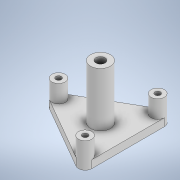
# Autodesk Inventor part: wheel_block
Saved by Autodesk Inventor 2021.3 (Build 253353010, 353A)
## iProperties
Created: 2021-11-06
Part Number: wheel_block
Material: Generic
Document SubType Name: Modeling
Designer: jesse
Density: 1 g/cm^3
Appearance: Default
Author: jesse
Autodesk Inventor part; units mm, degrees
ref_plane "YZ Plane" through (0, 0, 0) normal (1, 0, 0) x (0, 1, 0)
ref_plane "XZ Plane" through (0, 0, 0) normal (0, 1, 0) x (-1, 0, 0)
ref_plane "XY Plane" through (0, 0, 0) normal (0, 0, 1) x (1, 0, 0)
sketch "Sketch1" plane through (0, 0, 0) normal (0, 1, 0) x (-1, 0, 0)
  line L0 (27.1355, 0) -> (-13.5677, -23.5)
  line L1 (-13.5677, -23.5) -> (-13.5677, 23.5)
  line L2 (-13.5677, 23.5) -> (27.1355, 0)
  circle A0 centre (27.1355, 0) radius 1.8
  circle A1 centre (-13.5677, -23.5) radius 1.8
  circle A2 centre (-13.5677, 23.5) radius 1.8
  circle A3 centre (-13.5677, 23.5) radius 4.3
  circle A4 centre (-13.5677, -23.5) radius 4.3
  circle A5 centre (27.1355, 0) radius 4.3
  line L3 (37.2914, 0.8983) -> (-23.0689, -33.9507)
  line L4 (-17.8677, 35.8999) -> (-17.8677, -40.3839)
  line L5 (38.4842, -1.587) -> (-21.5839, 33.0933)
  point P0 (0, 0)
  point P1 (0, 0)
  point P2 (-11.4177, -27.2239)
  point P3 (29.2855, -3.7239)
  point P4 (29.2855, 3.7239)
  point P5 (-11.4177, 27.2239)
  point P6 (-17.8677, 23.5)
  point P7 (-17.8677, -23.5)
  dimension "d0" = 47
  dimension "d1" = 3.6
  dimension "d2" = 3.6
  dimension "d3" = 3.6
  dimension "d4" = 8.6
  dimension "d5" = 8.6
  dimension "d6" = 8.6
  constraints: 12 end point, 7 coincident, 6 centre point, 6 tangent, 7 other
  measures "d0" distance of L0.end L1.end
  measures "d1" diameter of A0
  measures "d2" diameter of A1
  measures "d3" diameter of A2
  measures "d4" diameter of A3
  measures "d5" diameter of A4
  measures "d6" diameter of A5
extrude "Extrusion1" add sketch "Sketch1" along normal blind 5 contours A0 L2 A5 L0 | L0 A5 L2 A0 | A5 L3 A4 L0 | L0 A4 L1 A3 L2 A5 | L2 A3 L5 A5 | A4 L1 A1 L0 | L0 A1 L1 A4 | A3 L1 A2 L2 | L2 A2 L1 A3 | A4 L4 A3 L1
sketch "Sketch2" plane through (0, 5, 0) normal (0, 1, 0) x (1, 0, 0)
  circle A0 centre (-27.1355, 0) radius 1.8 projected
  circle A1 centre (-27.1355, 0) radius 4.3
  circle A2 centre (13.5677, 23.5) radius 4.3
  circle A3 centre (13.5677, 23.5) radius 1.8 projected
  circle A4 centre (13.5677, -23.5) radius 1.8 projected
  line L0 (17.8677, -23.5) -> (17.8677, 23.5) projected
  circle A5 centre (13.5677, -23.5) radius 4.3
  point P0 (0, 0)
  dimension "d9" = 8.6
  dimension "d21" = 8.6
  dimension "d22" = 8.6
  constraints: 2 centre point, 2 coincident, 1 horizontal alignment, 2 other
  measures "d21" diameter of A1
  measures "d22" diameter of A5
extrude "Extrusion2" add sketch "Sketch2" along normal blind 11.5
sketch "Sketch3" plane through (0, 5, 0) normal (0, 1, 0) x (1, 0, 0)
  circle A0 centre (0, 0) radius 3
  circle A1 centre (0, 0) radius 6.45
  dimension "d12" = 6
  dimension "d13" = 12.9
  constraints: 2 centre point, 2 coincident
  measures "d12" diameter of A0
  measures "d13" diameter of A1
extrude "Extrusion3" add sketch "Sketch3" along normal blind 35
sketch "Sketch4" plane through (0, 0, 0) normal (0, -1, 0) x (1, 0, 0)
  circle A0 centre (0, 0) radius 3
  constraints: 1 centre point, 1 coincident
extrude "Extrusion4" cut sketch "Sketch4" against normal blind 36
sketch "Sketch5" plane through (0, 0, 0) normal (0, -1, 0) x (1, 0, 0)
  circle A0 centre (0, 0) radius 3 projected
  line L0 (-5, 2.8868) -> (0, 5.7735)
  line L1 (0, 5.7735) -> (5, 2.8868)
  line L2 (5, 2.8868) -> (5, -2.8868)
  line L3 (5, -2.8868) -> (0, -5.7735)
  line L4 (0, -5.7735) -> (-5, -2.8868)
  line L5 (-5, -2.8868) -> (-5, 2.8868)
  dimension "d18" = 10
  constraints: 12 end point, 1 coincident, 13 other
  measures "d18" distance between parallel lines of L3 L0
extrude "Extrusion5" cut sketch "Sketch5" against normal blind 4
equation "\"d21\" = d9"
equation "\"d22\" = d9"
body "Solid1"
